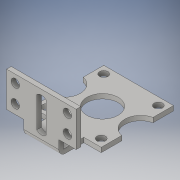
# Autodesk Inventor part: Motor Attach
Saved by Autodesk Inventor 2016 (Build 200138000, 138)
## iProperties
Created: 2017-09-12
Part Number: Motor Attach
Material: Generic
Document SubType Name: Modeling
Designer: student
Density: 1 g/cm^3
Appearance: Default
Author: student
Autodesk Inventor part; units mm, degrees
ref_plane "YZ Plane" through (0, 0, 0) normal (1, 0, 0) x (0, 1, 0)
ref_plane "XZ Plane" through (0, 0, 0) normal (0, 1, 0) x (-1, 0, 0)
ref_plane "XY Plane" through (0, 0, 0) normal (0, 0, 1) x (1, 0, 0)
sketch "Sketch1" plane through (0, 0, 0) normal (0, 0, 1) x (1, 0, 0)
  line L0 (21.971, 0) -> (21.971, 11.049)
  line L1 (21.971, 11.049) -> (0, 11.049)
  line L2 (0, 11.049) -> (0, 0)
  line L3 (5.4483, 0) -> (5.4483, -4.7752)
  line L4 (5.4483, -4.7752) -> (16.5227, -4.7752)
  line L5 (16.5227, -4.7752) -> (16.5227, 0)
  line L6 (21.971, 0) -> (16.5227, 0)
  line L7 (0, 0) -> (5.4483, 0)
  arc A0 (12.4587, 8.9011) -> (9.5123, 8.8875) centre (10.9928, 7.313) ccw
  arc A1 (9.5123, -0.8104) -> (12.4587, -0.7909) centre (10.9765, 0.5527) ccw
  line L8 (9.5123, 8.8875) -> (9.5123, -0.8104)
  line L9 (12.4587, 8.9011) -> (12.4587, -0.7909)
  circle A2 centre (2.7664, 8.558) radius 1.3335
  circle A3 centre (2.7453, 2.9191) radius 1.3341
  circle A4 centre (19.2468, 8.558) radius 1.3335
  circle A5 centre (19.2468, 2.9191) radius 1.3335
  point P0 (10.9855, 0)
  dimension "d0" = 21.971
  dimension "d1" = 11.049
  dimension "d2" = 5.5372
  dimension "d3" = 5.5372
  dimension "d4" = 4.7752
  dimension "d9" = 2.667
  dimension "d10" = 2.667
  constraints: 20 end point, 6 centre point, 4 point on circle, 3 perpendicular, 3 vertical, 1 parallel
  measures "d0" distance of L1.end L0.end
  measures "d1" distance of L0.start L0.end
  measures "d2" distance of point (10.985, 0) L3.start
  measures "d3" distance of point (10.985, 0) L5.end
  measures "d4" distance of L3.start L3.end
  measures "d9" diameter of A2
  measures "d10" diameter of A4
extrude "Extrusion1" add sketch "Sketch1" along normal blind 1.4732
sketch "Sketch2" plane through (5.4483, -4.7752, 0) normal (0, -1, 0) x (1, 0, 0)
  line L0 (0, 1.4732) -> (11.0744, 1.4732)
  line L1 (11.0744, 1.4732) -> (11.0744, -6.4262)
  line L2 (0, -6.4262) -> (0, 1.4732)
  line L3 (0, -6.4262) -> (-5.4864, -6.4262)
  line L4 (11.0744, -6.4262) -> (16.5608, -6.4262)
  line L5 (-5.4864, -29.2862) -> (16.5608, -29.2862)
  circle A0 centre (5.5372, -17.8562) radius 4.953
  arc A1 (-5.4864, -22.8092) -> (-5.4864, -12.9032) centre (-6.5684, -17.8562) ccw
  arc A2 (16.5608, -12.9032) -> (16.5608, -22.8092) centre (17.6428, -17.8562) ccw
  line L6 (-5.4864, -6.4262) -> (-5.4864, -12.9032)
  line L7 (-5.4864, -22.8092) -> (-5.4864, -29.2862)
  line L8 (16.5608, -29.2862) -> (16.5608, -22.8092)
  line L9 (16.5608, -12.9032) -> (16.5608, -6.4262)
  line L10 (16.5608, -6.4262) -> (15.494, -6.4262)
  line L11 (16.5608, -7.493) -> (16.5608, -6.4262)
  circle A3 centre (14.1605, -8.8265) radius 1.3335
  circle A4 centre (14.1605, -26.8859) radius 1.3335
  circle A5 centre (-3.0861, -8.8265) radius 1.3335
  circle A6 centre (-3.0861, -26.8859) radius 1.3335
  constraints: 24 end point, 7 centre point, 4 point on circle, 3 horizontal, 3 perpendicular, 2 vertical, 1 parallel
extrude "Extrusion2" add sketch "Sketch2" against normal blind 1.4732
fillet "Fillet1" radius 2.032 1 edges at (10.9855, -4.7752, 1.4732)
body "Solid1"
